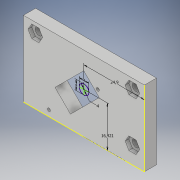
# Autodesk Inventor part: 30_CUBE_penSIM_DMD_Holder
Saved by Autodesk Inventor 2019 (Build 230136000, 136)
## iProperties
Created: 2020-08-18
Part Number: 30_CUBE_penSIM_DMD_Holder
Material: Generic
Document SubType Name: Modeling
Designer: wanghaoran
Density: 1 g/cm^3
Appearance: Default
Author: wanghaoran
Autodesk Inventor part; units mm, degrees
ref_plane "YZ Plane" through (0, 0, 0) normal (1, 0, 0) x (0, 1, 0)
ref_plane "XZ Plane" through (0, 0, 0) normal (0, 1, 0) x (-1, 0, 0)
ref_plane "XY Plane" through (0, 0, 0) normal (0, 0, 1) x (1, 0, 0)
sketch "Sketch1" plane through (0, 0, 0) normal (0, 0, 1) x (1, 0, 0)
  line L0 (0, 0) -> (49.8, 0)
  line L1 (49.8, 0) -> (49.8, 30.921)
  line L2 (49.8, 30.921) -> (0, 30.921)
  line L3 (0, 30.921) -> (0, 0)
  dimension "d0" = 49.8
  dimension "d1" = 30.921
  constraints: 8 end point, 2 parallel, 1 horizontal, 1 perpendicular
  measures "d0" distance of L2.end L1.end
  measures "d1" distance of L1.end L0.end
extrude "Extrusion1" add sketch "Sketch1" along normal blind 5
sketch "Sketch3" plane through (0, 0, 5) normal (0, 0, 1) x (1, 0, 0)
  line L0 (0, 0) -> (49.8, 0) projected
  line L1 (24.9, 0) -> (41.821, 0) construction
  line L2 (49.8, 0) -> (49.8, 30.921) projected
  line L3 (22.9, 16.921) -> (26.9, 16.921)
  line L4 (24.9, 14.921) -> (24.9, 18.921)
  circle A0 centre (24.9, 16.921) radius 2
  dimension "d22" = 4
  dimension "d23" = 4
  dimension "d24" = 4
  dimension "d25" = 16.921
  dimension "d26" = 24.9
  constraints: 6 end point, 1 centre point, 1 horizontal, 1 midpoint, 1 perpendicular
  measures "d22" distance of L3.start L3.end
  measures "d23" distance of L4.start L4.end
  measures "d24" diameter of A0
  measures "d25" distance from line of L0 A0.centre
  measures "d26" distance from line of L2 A0.centre
sketch "Sketch4" plane through (0, 0, 5) normal (0, 0, 1) x (1, 0, 0)
  line L0 (0, 0) -> (49.8, 0) projected
  line L1 (0, 0) -> (7.1085, 7.1085)
  line L2 (0, 0) -> (10.053, 0) construction
  line L3 (17.8214, 5.3223) -> (45.7841, 5.3223) construction
  line L4 (22.1418, 11.0415) -> (25.8541, 14.7538)
  line L5 (25.8541, 14.7538) -> (23.7328, 16.8751)
  line L6 (23.7328, 16.8751) -> (20.0205, 13.1628)
  line L7 (20.0205, 13.1628) -> (22.1418, 11.0415)
  line L8 (16.6871, 14.6491) -> (21.9371, 14.6491) construction
  line L9 (20.0205, 13.1628) -> (25.8541, 14.7538)
  line L10 (23.7328, 16.8751) -> (22.1418, 11.0415)
  line L11 (22.9373, 13.9583) -> (23.9979, 12.8976)
  line L12 (22.9, 16.921) -> (26.9, 16.921) projected
  line L13 (24.9, 14.921) -> (24.9, 18.921) projected
  circle A0 centre (24.9, 16.921) radius 2 projected
  line L14 (22.8984, 10.2849) -> (26.6107, 13.9972)
  line L15 (6.9567, 4.2426) -> (27.8163, 25.1023)
  line L16 (32.6954, 20.2233) -> (64.1581, 20.2233) construction
  circle A1 centre (30.6448, 19.799) radius 0.75
  circle A2 centre (10.4922, 2.4749) radius 0.75
  line L17 (31.2069, 17.1792) -> (24.8429, 23.5431)
  line L18 (12.9989, 11.6991) -> (19.3629, 5.3351)
  line L19 (26.6107, 13.9972) -> (32.7661, 20.1525)
  line L20 (20.6107, 13.9972) -> (29.3157, 13.9972) construction
  line L21 (32.7661, 20.1525) -> (11.9064, -0.7071)
  line L22 (11.9064, -0.7071) -> (6.9567, 4.2426)
  line L23 (27.8163, 25.1023) -> (32.7661, 20.1525)
  line L24 (29.0217, 22.4081) -> (58.5217, 22.4081) construction
  line L25 (12.9989, 11.6991) -> (24.8429, 23.5431)
  line L26 (31.2069, 17.1792) -> (19.3629, 5.3351)
  line L27 (14.162, 1.5485) -> (11.9064, -0.7071)
  line L28 (10.9064, -0.7071) -> (14.0963, -0.7071) construction
  line L29 (10.8458, 2.8284) -> (10.4922, 2.4749)
  line L30 (10.8458, 2.8284) -> (11.3458, 2.8284) construction
  line L31 (10.9064, -0.7071) -> (11.9064, -0.7071)
  circle A3 centre (30.6448, 19.799) radius 0.6
  circle A4 centre (10.4922, 2.4749) radius 0.6
  point P0 (25.55, 22.836)
  point P1 (13.706, 10.992)
  dimension "d27" = 10.053
  dimension "d28" = 45
  dimension "d32" = 5.25
  dimension "d33" = 45
  dimension "d34" = 3
  dimension "d36" = 1.07
  dimension "d40" = 1.5
  dimension "d43" = 1.5
  dimension "d46" = 5.5
  dimension "d47" = 6
  dimension "d51" = 8.705
  dimension "d52" = 45
  dimension "d53" = 29.5
  dimension "d54" = 135
  dimension "d55" = 7
  dimension "d56" = 3.75
  dimension "d57" = 1
  dimension "d58" = 1
  dimension "d59" = 2.93
  dimension "d60" = 1.25
  dimension "d61" = 1.75
  dimension "d97" = 135
  dimension "d98" = 0.5
  dimension "d99" = 135
  dimension "d101" = 1
  dimension "d102" = 1.2
  dimension "d103" = 1.2
  constraints: 58 end point, 9 horizontal, 7 parallel, 6 equal length, 4 centre point, 4 point on line, 2 coincident, 2 midpoint, 2 perpendicular
  measures "d27" distance of L0.start L1.end
  measures "d28" angle of L2 L1
  measures "d32" distance of L4.start L4.end
  measures "d33" angle of L8 L4
  measures "d34" distance of L5.end L4.end
  measures "d36" distance between parallel lines of L4 L14
  measures "d40" diameter of A1
  measures "d43" diameter of A2
  measures "d46" distance between parallel lines of L5 L17
  measures "d47" distance between parallel lines of L7 L18
  measures "d51" distance of L14.end L19.end
  measures "d52" angle of L20 L19
  measures "d53" distance of L19.end L21.end
  measures "d54" angle of L21 L24
  measures "d55" distance of L21.end L22.end
  measures "d56" distance from line of L15 A2.centre
  measures "d57" distance between parallel lines of L15 L25
  measures "d58" distance between parallel lines of L21 L26
  measures "d59" distance between parallel lines of L15 L6
  measures "d60" distance from line of L21 A1.centre
  measures "d61" distance from line of L23 A1.centre
  measures "d97" angle of L27 L28
  measures "d98" distance of L29.start L29.end
  measures "d99" angle of L29 L30
  measures "d101" distance of L31.start L31.end
  measures "d102" diameter of A3
  measures "d103" diameter of A4
extrude "Extrusion3" cut sketch "Sketch4" against normal blind 5 contours L18 L25 L17 L15 | L15 L17 L19 L14 L21 L18 | L21 L14 L19 L17 L26 L18 | L10 L11 L4 | L7 L9 L10 | L11 L9 L4 | L6 A0 L10 L9 | L10 A0 L5 L9 | A0 L12 L13 L5 L6 | L6 L10 A0 | L10 L5 L13 A0 | A0 L13 L5 | L5 L13 L12 A0 | A0 L13 L12 | L12 L13 A0 | A3 | A4
sketch "Sketch5" plane through (0, 0, 5) normal (0, 0, 1) x (1, 0, 0)
  circle A0 centre (4.9, 26.921) radius 1.55
  circle A1 centre (44.9, 7) radius 1.55
  circle A2 centre (44.9, 26.921) radius 1.55
  line L0 (0, 30.921) -> (0, 0) projected
  line L1 (49.8, 30.921) -> (0, 30.921) projected
  line L2 (49.8, 0) -> (49.8, 30.921) projected
  line L3 (0, 0) -> (49.8, 0) projected
  dimension "d62" = 3.1
  dimension "d63" = 3.1
  dimension "d64" = 3.1
  dimension "d65" = 4.9
  dimension "d66" = 4
  dimension "d67" = 4.9
  dimension "d68" = 4
  dimension "d69" = 4.9
  dimension "d70" = 7
  constraints: 3 centre point
  measures "d62" diameter of A0
  measures "d63" diameter of A1
  measures "d64" diameter of A2
  measures "d65" distance from line of L0 A0.centre
  measures "d66" distance from line of L1 A0.centre
  measures "d67" distance from line of L2 A2.centre
  measures "d68" distance from line of L1 A2.centre
  measures "d69" distance from line of L2 A1.centre
  measures "d70" distance from line of L3 A1.centre
extrude "Extrusion4" cut sketch "Sketch5" against normal blind 5 contours A0 | A1 | A2
sketch "Sketch6" plane through (0, 0, 5) normal (0, 0, 1) x (1, 0, 0)
  circle A0 centre (4.9, 26.921) radius 1.55 projected
  line L0 (2.15, 29.671) -> (7.65, 24.171) construction
  line L1 (7.65, 29.671) -> (2.15, 24.171) construction
  line L2 (3.3975, 24.3186) -> (1.895, 26.921)
  line L3 (1.895, 26.921) -> (3.3975, 29.5234)
  line L4 (3.3975, 29.5234) -> (6.4025, 29.5234)
  line L5 (6.4025, 29.5234) -> (7.905, 26.921)
  line L6 (7.905, 26.921) -> (6.4025, 24.3186)
  line L7 (6.4025, 24.3186) -> (3.3975, 24.3186)
  line L8 (43.3975, 29.5234) -> (46.4025, 29.5234)
  line L9 (41.895, 26.921) -> (43.3975, 29.5234)
  line L10 (43.3975, 24.3186) -> (41.895, 26.921)
  line L11 (46.4025, 24.3186) -> (43.3975, 24.3186)
  line L12 (47.905, 26.921) -> (46.4025, 24.3186)
  line L13 (46.4025, 29.5234) -> (47.905, 26.921)
  line L14 (44.9, 26.921) -> (44.9, 16.921)
  line L15 (43.3975, 4.3976) -> (41.895, 7)
  line L16 (41.895, 7) -> (43.3975, 9.6024)
  line L17 (43.3975, 9.6024) -> (46.4025, 9.6024)
  line L18 (46.4025, 9.6024) -> (47.905, 7)
  line L19 (47.905, 7) -> (46.4025, 4.3976)
  line L20 (46.4025, 4.3976) -> (43.3975, 4.3976)
  point P0 (0, 0)
  point P1 (44.9, 7)
  dimension "d73" = 5.5
  dimension "d74" = 5.5
  dimension "d81" = 6.01
  dimension "d84" = 40
  dimension "d89" = 10
  dimension "d92" = 19.921
  constraints: 42 end point, 2 midpoint, 2 vertical, 1 coincident, 1 collinear, 1 horizontal, 36 other
  measures "d73" distance of L0.end L1.end
  measures "d74" distance of L1.start L0.end
  measures "d81" distance of L5.end L2.end
  measures "d84" distance of L3.end L8.start
  measures "d89" distance of L14.start L14.end
  measures "d92" distance of L10.start L15.start
extrude "Extrusion5" cut sketch "Sketch6" against normal blind 1.5
body "Solid1"
